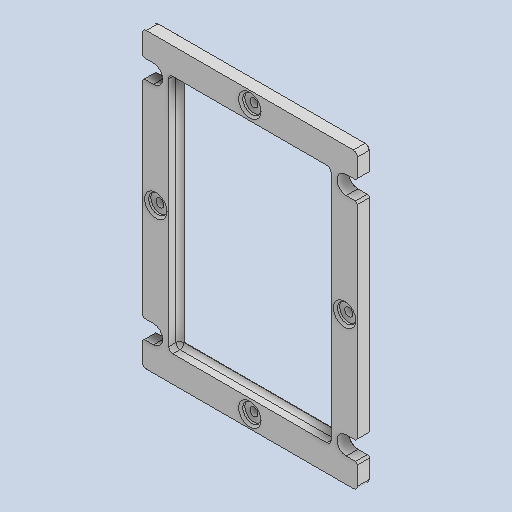
# Autodesk Inventor part: BatteryHolder
Saved by Autodesk Inventor 2022 (Build 260153000, 153)
## iProperties
Created: 2021-02-16
Part Number: BatteryHolder
Material: Generic
Document SubType Name: Modeling
Designer: Viktor
Density: 1 g/cm^3
Appearance: Default
Author: Viktor
## iProperties of the stored document _3DPrint.ipt
Created: 2021-02-17
Part Number: _3DPrint
Material: Generic
Document SubType Name: Modeling
Designer: Viktor
Density: 1 g/cm^3
Appearance: Default
Author: Viktor
Autodesk Inventor part; units mm, degrees
ref_plane "YZ Plane" through (0, 0, 0) normal (1, 0, 0) x (0, 1, 0)
ref_plane "XZ Plane" through (0, 0, 0) normal (0, 1, 0) x (-1, 0, 0)
ref_plane "XY Plane" through (0, 0, 0) normal (0, 0, 1) x (1, 0, 0)
sketch "Sketch1" plane through (0, 0, 0) normal (0, 0, 1) x (1, 0, 0)
  line L0 (-39.6, -58.6) -> (39.6, -58.6)
  line L1 (39.6, -58.6) -> (39.6, 58.6)
  line L2 (39.6, 58.6) -> (-39.6, 58.6)
  line L3 (-39.6, 58.6) -> (-39.6, -58.6)
  line L4 (-39.6, -58.6) -> (39.6, 58.6) construction
  line L5 (39.6, -58.6) -> (-39.6, 58.6) construction
  line L6 (-52.5, -71.5) -> (52.5, -71.5)
  line L7 (52.5, -71.5) -> (52.5, 71.5)
  line L8 (52.5, 71.5) -> (-52.5, 71.5)
  line L9 (-52.5, 71.5) -> (-52.5, -71.5)
  line L10 (-52.5, -71.5) -> (52.5, 71.5) construction
  line L11 (52.5, -71.5) -> (-52.5, 71.5) construction
  line L12 (0, 100.1) -> (0, -100.1) projected
  line L13 (-73.5, 0) -> (73.5, 0) projected
  circle A0 centre (-45.85, 0) radius 2
  circle A1 centre (46.25, 0) radius 2
  circle A2 centre (0, 65.25) radius 2
  circle A3 centre (0, -65.25) radius 2
  point P0 (0, 0)
  dimension "d0" = 79.2
  dimension "d1" = 117.2
  dimension "d2" = 105
  dimension "d4" = 12.9
  dimension "d6" = 6.25
  dimension "d7" = 6.25
  dimension "d8" = 6.25
  dimension "d9" = 6.25
  dimension "d10" = 4
  dimension "d11" = 4
  dimension "d12" = 4
  dimension "d40" = 143
  dimension "d41" = 4
  constraints: 24 end point, 4 centre point, 4 midpoint, 4 parallel, 4 point on line, 2 horizontal, 2 perpendicular
  measures "d0" distance between parallel lines of L1 L3
  measures "d1" distance of L0.end L1.end
  measures "d2" distance between parallel lines of L7 L9
  measures "d4" distance between parallel lines of L7 L1
  measures "d6" distance from line of A0.centre L3
  measures "d7" distance from line of L7 A1.centre
  measures "d8" distance from line of L6 A3.centre
  measures "d9" distance from line of L8 A2.centre
  measures "d10" diameter of A0
  measures "d11" diameter of A2
  measures "d12" diameter of A1
  measures "d40" distance between parallel lines of L6 L8
  measures "d41" diameter of A3
extrude "Extrusion1" add sketch "Sketch1" along normal blind 6 contours L0 L12 A3 L6 L9 L13 A0 L3 | L0 L1 L13 A1 L7 L6 L12 A3 | L13 A0 L9 L8 L12 A2 L2 L3 | L1 L2 L12 A2 L8 L7 L13 A1
fillet "Fillet1" radius 2 8 edges at (-39.6, 58.6, 3) (39.6, 58.6, 3) (39.6, -58.6, 3) (-39.6, -58.6, 3) (52.5, 71.5, 3) (-52.5, 71.5, 3) (-52.5, -71.5, 3) (52.5, -71.5, 3)
sketch "Sketch2" plane through (0, 0, 6) normal (0, 0, 1) x (1, 0, 0)
  circle A0 centre (0, 65.25) radius 2 projected
  circle A1 centre (46.25, 0) radius 2 projected
  circle A2 centre (0, -65.25) radius 2 projected
  circle A3 centre (-45.85, 0) radius 2 projected
  circle A4 centre (0, 65.25) radius 4.5
  circle A5 centre (46.25, 0) radius 4.5
  circle A6 centre (0, -65.25) radius 4.5
  circle A7 centre (-45.85, 0) radius 4.5
  point P0 (0, 0)
  dimension "d16" = 9
  dimension "d17" = 9
  dimension "d18" = 9
  dimension "d19" = 9
  constraints: 4 centre point
  measures "d16" diameter of A4
  measures "d17" diameter of A5
  measures "d18" diameter of A7
  measures "d19" diameter of A6
extrude "Extrusion2" cut sketch "Sketch2" against normal blind 2
chamfer "Chamfer1" distance 1 angle 45 4 edges at (-4.5, 65.25, 6) (-50.35, 0, 6) (41.75, 0, 6) (-4.5, -65.25, 6)
sketch "Sketch3" plane through (0, 0, 6) normal (0, 0, 1) x (1, 0, 0)
  circle A0 centre (-47, -55) radius 4.5
  line L0 (-73.5, 0) -> (73.5, 0) construction
  line L1 (0, 100.1) -> (0, -100.1) construction
  line L2 (-47, -50.5) -> (-52.5, -50.5)
  line L3 (-52.5, 69.5) -> (-52.5, -69.5) construction
  line L4 (-52.5, -50.5) -> (-52.5, -59.5)
  line L5 (-52.5, -59.5) -> (-47, -59.5)
  circle A1 centre (47, -55) radius 4.5
  line L6 (47, -50.5) -> (52.5, -50.5)
  line L7 (52.5, -50.5) -> (52.5, -59.5)
  line L8 (52.5, -59.5) -> (47, -59.5)
  circle A2 centre (-47, 55) radius 4.5
  line L9 (-47, 50.5) -> (-52.5, 50.5)
  line L10 (-52.5, 50.5) -> (-52.5, 59.5)
  line L11 (-52.5, 59.5) -> (-47, 59.5)
  circle A3 centre (47, 55) radius 4.5
  line L12 (47, 50.5) -> (52.5, 50.5)
  line L13 (52.5, 50.5) -> (52.5, 59.5)
  line L14 (52.5, 59.5) -> (47, 59.5)
  point P0 (0, 0)
  dimension "d25" = 9
  dimension "d26" = 55
  dimension "d27" = 47
  constraints: 24 end point, 15 symmetric about line, 8 point on circle, 4 centre point, 2 point on line, 1 horizontal, 1 perpendicular, 3 other
  measures "d25" diameter of A0
  measures "d26" distance from line of L0 A0.centre
  measures "d27" distance from line of L1 A0.centre
extrude "Extrusion3" cut sketch "Sketch3" against normal through all
chamfer "Chamfer2" distance 1 angle 45 8 edges at (-52.5, -50.5, 3) (-52.5, -59.5, 3) (52.5, -59.5, 3) (52.5, -50.5, 3) (52.5, 59.5, 3) (52.5, 50.5, 3) (-52.5, 59.5, 3) (-52.5, 50.5, 3)
sketch "Sketch4" plane through (0, 0, 0) normal (0, 0, -1) x (-1, 0, 0)
  line L0 (37.6, 58.6) -> (-37.6, 58.6) projected
  arc A0 (39.6, 56.6) -> (37.6, 58.6) centre (37.6, 56.6) ccw projected
  line L1 (39.6, -56.6) -> (39.6, 56.6) projected
  arc A1 (37.6, -58.6) -> (39.6, -56.6) centre (37.6, -56.6) ccw projected
  line L2 (-37.6, -58.6) -> (37.6, -58.6) projected
  arc A2 (-39.6, -56.6) -> (-37.6, -58.6) centre (-37.6, -56.6) ccw projected
  line L3 (-39.6, 56.6) -> (-39.6, -56.6) projected
  arc A3 (-37.6, 58.6) -> (-39.6, 56.6) centre (-37.6, 56.6) ccw projected
  line L4 (-37.6, 56.6) -> (37.6, 56.6)
  line L5 (37.6, 56.6) -> (37.6, -56.6)
  line L6 (37.6, -56.6) -> (-37.6, -56.6)
  line L7 (-37.6, -56.6) -> (-37.6, 56.6)
  point P0 (0, 0)
  point P1 (37.6, 56.6)
  point P2 (-37.6, -56.6)
  dimension "d33" = 2
  constraints: 8 end point, 23 other
  measures "d33" distance between parallel lines of L0 L4
extrude "Extrusion4" add sketch "Sketch4" against normal blind 0.5
fillet "Fillet2" radius 2 8 edges at (39.0142, 58.0142, 0.5) (39.6, 0, 0.5) (39.0142, -58.0142, 0.5) (0, -58.6, 0.5) (-39.0142, -58.0142, 0.5) (-39.6, 0, 0.5) (-39.0142, 58.0142, 0.5) (0, 58.6, 0.5)
chamfer "Chamfer3" distance 0.3 angle 45 28 edges at (0, 71.5, 0) (-51.9142, 70.9142, 0) (-52.5, 65, 0) (51.9142, 70.9142, 0) (52.5, 65, 0) (42.5, 55, 0) (49.25, 50.5, 0) (49.25, 59.5, 0) (52.5, 0, 0) (42.5, -55, 0) (49.25, -59.5, 0) (49.25, -50.5, 0) (52.5, -65, 0) (51.9142, -70.9142, 0) (0, -71.5, 0) (-51.9142, -70.9142, 0) (-52.5, -65, 0) (-42.5, -55, 0) (-49.25, -50.5, 0) (-49.25, -59.5, 0) (-52.5, 0, 0) (-49.25, 59.5, 0) (-42.5, 55, 0) (-49.25, 50.5, 0) (0, 56.6, 0) (-37.6, 0, 0) (37.6, 0, 0) (0, -56.6, 0)
equation "\"d7\" = d6"
equation "\"d8\" = d6"
equation "\"d9\" = d6"
equation "\"d11\" = d10"
equation "\"d12\" = d10"
equation "\"d41\" = d11"
equation "\"d17\" = d16"
equation "\"d18\" = d16"
equation "\"d19\" = d18"
body "Solid1"
